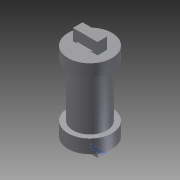
# Autodesk Inventor part: LargeSmallGearAxis
Saved by Autodesk Inventor 2012 (Build 160160000, 160)
## iProperties
Created: 2011-10-22
Part Number: LargeSmallGearAxis
Material: Default
Document SubType Name: Modeling
Designer: KuttaA
Density: 1 g/cm^3
Mass: 0.137107 g
Surface Area: 2.1959 cm^2
Volume: 0.137107 cm^3
Author: KuttaA
Autodesk Inventor part; units mm, degrees
ref_plane "YZ Plane" through (0, 0, 0) normal (1, 0, 0) x (0, 1, 0)
ref_plane "XZ Plane" through (0, 0, 0) normal (0, 1, 0) x (-1, 0, 0)
ref_plane "XY Plane" through (0, 0, 0) normal (0, 0, 1) x (1, 0, 0)
sketch "Sketch1" plane through (0, 0, 0) normal (0, 0, 1) x (1, 0, 0)
  circle A0 centre (0, 0) radius 1.65 projected
  circle A1 centre (0, 0) radius 1.35
  point P0 (0, 0)
  dimension "d21" = 2.7
  constraints: 1 centre point, 1 coincident
  measures "d21" diameter of A1
extrude "Extrusion1" add sketch "Sketch1" along normal blind 5 and the other way blind 15 contours A1
sketch "Sketch2" plane through (0, 0, 5) normal (0, 0, 1) x (1, 0, 0)
  circle A0 centre (0, 0) radius 1.35 projected
  line L0 (-0.9546, 0.9546) -> (0.9546, 0.9546)
  line L1 (0.9546, 0.9546) -> (0.9546, -0.9546)
  line L2 (0.9546, -0.9546) -> (-0.9546, -0.9546)
  line L3 (-0.9546, -0.9546) -> (-0.9546, 0.9546)
  circle A1 centre (0, 0) radius 1.35 projected
  point P0 (0, 0)
  constraints: 8 end point, 4 point on circle, 2 parallel, 2 perpendicular, 1 horizontal
extrude "Extrusion2" cut sketch "Sketch2" against normal blind 2 contours A0 L1 | L0 A0 | A0 L2 | L3 A0
sketch "Sketch3" plane through (0, 0, 3) normal (0, 0, 1) x (1, 0, 0)
  arc A0 (-0.9546, 0.9546) -> (-0.9546, -0.9546) centre (0, 0) ccw projected
  arc A1 (0.9546, 0.9546) -> (-0.9546, 0.9546) centre (0, 0) ccw projected
  arc A2 (0.9546, -0.9546) -> (0.9546, 0.9546) centre (0, 0) ccw projected
  arc A3 (-0.9546, -0.9546) -> (0.9546, -0.9546) centre (0, 0) ccw projected
  arc A4 (-0.9546, 0.9546) -> (-0.9546, -0.9546) centre (0, 0) ccw projected
  circle A5 centre (0, 0) radius 1.35 projected
  circle A6 centre (0, 0) radius 1.9092
  point P0 (0, 0)
  constraints: 1 centre point, 1 coincident
extrude "Extrusion3" add sketch "Sketch3" against normal blind 2.7
sketch "Sketch4" plane through (0, 0, -15) normal (0, 0, -1) x (-1, 0, 0)
  circle A0 centre (0, 0) radius 1.35 projected
  circle A1 centre (0, 0) radius 1.35 projected
  circle A2 centre (0, 0) radius 1.9092 projected
  line L0 (-0.9546, -0.9546) -> (-0.9546, 0.9546) projected
  line L1 (0.9546, -0.9546) -> (-0.9546, -0.9546) projected
  line L2 (0.9546, 0.9546) -> (0.9546, -0.9546) projected
  line L3 (-0.9546, 0.9546) -> (0.9546, 0.9546) projected
extrude "Extrusion4" cut sketch "Sketch4" against normal blind 2 contours A0 L2 | L3 A0 | A0 L1 | L0 A0
sketch "Sketch5" plane through (0, 0, -13) normal (0, 0, -1) x (-1, 0, 0)
  circle A0 centre (0, 0) radius 1.9092 projected
  point P0 (0, 0)
extrude "Extrusion5" add sketch "Sketch5" against normal blind 2.7
sketch "Sketch7" plane through (-0.9546, -0.9546, -15) normal (0, -1, 0) x (1, 0, 0)
  line L0 (1.9092, 2) -> (0, 2) construction
  line L1 (0, 0) -> (0, 2) construction
  line L2 (1.9092, 2) -> (1.9092, 0) construction
  line L3 (-1.4999, 2) -> (3.4091, 2)
  line L4 (3.4091, 2) -> (3.4091, 0)
  line L5 (3.4091, 0) -> (-1.4999, 0)
  line L6 (-1.4999, 0) -> (-1.4999, 2)
  line L7 (0.9546, 19.9961) -> (0.9546, 0)
  line L8 (0.9546, 9.998) -> (8.9961, 9.998)
  line L9 (-1.4999, 17.9961) -> (3.4091, 17.9961)
  line L10 (3.4091, 17.9961) -> (3.4091, 19.9961)
  line L11 (3.4091, 19.9961) -> (-1.4999, 19.9961)
  line L12 (-1.4999, 19.9961) -> (-1.4999, 17.9961)
  point P0 (0.9546, 15)
  dimension "d13" = 4.909
  dimension "d14" = 1.4999
  dimension "d15" = 1.9092
  dimension "d16" = 2
  dimension "d17" = 2
  dimension "d18" = 0
  constraints: 20 end point, 4 symmetric about line, 2 midpoint, 2 parallel, 2 perpendicular, 1 horizontal
  measures "d13" distance of L4.end L5.end
  measures "d14" distance between parallel lines of L4 L2
  measures "d15" distance between parallel lines of L2 L1
  measures "d16" distance of L1.start L0.end
  measures "d17" distance between parallel lines of L3 L5
  measures "d18" distance between parallel lines of L0 L3
extrude "Extrusion6" add sketch "Sketch7" against normal up to surface (1.9092 mm away)
sketch "Sketch8" plane through (0, 0, -10.3) normal (0, 0, 1) x (1, 0, 0)
  circle A0 centre (0, 0) radius 1.35 projected
  circle A1 centre (0, 0) radius 3.375
  dimension "d22" = 2.7
  dimension "d23" = 6.75
  constraints: 1 centre point, 1 coincident
  measures "d22" diameter of A0
  measures "d23" diameter of A1
extrude "Extrusion7" add sketch "Sketch8" along normal up to surface (10.6 mm away)
sketch "Sketch9" plane through (0, 0, -10.3) normal (0, 0, -1) x (-1, 0, 0)
  circle A0 centre (0, 0) radius 3.375 projected
  circle A1 centre (0, 0) radius 1.9092 projected
  circle A2 centre (0, 0) radius 4.375
  dimension "d26" = 1
  constraints: 1 centre point, 1 coincident
  measures "d26" radial gap between concentric circles of A2 A0
extrude "Extrusion8" add sketch "Sketch9" along normal up to surface (2.7 mm away) contours A0 | A2
sketch "Sketch10" plane through (0, 0, 0.3) normal (0, 0, 1) x (1, 0, 0)
  circle A0 centre (0, 0) radius 1.9092 projected
  circle A1 centre (0, 0) radius 4.375 projected
extrude "Extrusion9" add sketch "Sketch10" along normal up to surface (2.7 mm away)
sketch "Sketch12" plane through (0, 0, 3) normal (0, 0, 1) x (1, 0, 0)
  circle A0 centre (0, 0) radius 4.375 projected
  line L0 (2.4545, -0.9546) -> (-2.4545, -0.9546) projected
  line L1 (-2.4545, 0.9546) -> (-2.4545, -0.9546) projected
  line L2 (2.4545, 0.9546) -> (-2.4545, 0.9546) projected
  line L3 (2.4545, -0.9546) -> (2.4545, 0.9546) projected
extrude "Extrusion11" cut sketch "Sketch12" against normal blind 0.3
sketch "Sketch13" plane through (0, 0, -13) normal (0, 0, -1) x (-1, 0, 0)
  circle A0 centre (0, 0) radius 4.375 projected
  line L0 (-2.4545, 0.9546) -> (2.4545, 0.9546) projected
  line L1 (2.4545, -0.9546) -> (2.4545, 0.9546) projected
  line L2 (-2.4545, -0.9546) -> (2.4545, -0.9546) projected
  line L3 (-2.4545, -0.9546) -> (-2.4545, 0.9546) projected
extrude "Extrusion12" cut sketch "Sketch13" against normal blind 0.3
equation "\"d14\" = -0.5 * d15 + 0.5 * d13"
equation "\"d23\" = 2.5 * d22"
body "Solid1"
